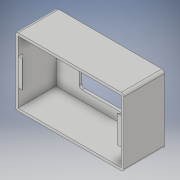
# Autodesk Inventor part: spodok
Saved by Autodesk Inventor 2019 (Build 230136000, 136)
## iProperties
Created: 2021-04-22
Part Number: spodok
Material: Všeobecné
Document SubType Name: Modeling
Designer: miko flosso
Density: 1 g/cm^3
Appearance: Výchozí
Author: miko flosso
Autodesk Inventor part; units mm, degrees
ref_plane "YZ Plane" through (0, 0, 0) normal (1, 0, 0) x (0, 1, 0)
ref_plane "XZ Plane" through (0, 0, 0) normal (0, 1, 0) x (-1, 0, 0)
sketch "Náčrt3" plane through (0, 0, 0) normal (0, 0, 1) x (1, 0, 0)
  line L0 (2, 0) -> (78, 0)
  line L1 (80, -2) -> (80, -48)
  line L2 (78, -50) -> (2, -50)
  line L3 (0, -48) -> (0, -2)
  arc A0 (2, 0) -> (0, -2) centre (2, -2) ccw
  arc A1 (0, -48) -> (2, -50) centre (2, -48) ccw
  arc A2 (80, -2) -> (78, 0) centre (78, -2) ccw
  arc A3 (78, -50) -> (80, -48) centre (78, -48) ccw
  point P0 (0, 0)
  point P1 (80, -50)
  point P2 (80, 0)
  point P3 (0, -50)
  dimension "d4" = 80
  dimension "d5" = 50
  dimension "d6" = 2
  constraints: 8 end point, 8 point on circle, 8 point on line, 8 tangent, 4 centre point, 3 equal radius, 2 parallel, 1 horizontal, 1 perpendicular
  measures "d4" distance of point (80, -50) point (0, -50)
  measures "d5" distance of point (80, 0) point (80, -50)
  measures "d6" radius of A0
extrude "Vysunutí2" add sketch "Náčrt3" along normal blind 30
shell "Skořepina1" thickness 2 removed faces 1 at (27.3333, -16.6667, 30)
sketch "Náčrt4" plane through (2, -48, 30) normal (1, 0, 0) x (0, 0, -1)
  line L0 (0.0823, 33) -> (3.0823, 33)
  line L1 (3.0823, 33) -> (3.0823, 13)
  line L2 (3.0823, 13) -> (0.0823, 13)
  line L3 (0.0823, 13) -> (0.0823, 33)
  point P0 (30, 48)
  dimension "d10" = 3
  dimension "d11" = 20
  dimension "d12" = 15
  constraints: 8 end point, 2 parallel, 1 horizontal, 1 perpendicular
  measures "d10" distance of L1.end L2.end
  measures "d11" distance of L0.end L1.end
  measures "d12" distance from line of point (30, 48) L0
extrude "Vysunutí3" add sketch "Náčrt4" along normal blind 3
chamfer "Zkosení1" distance 2.5 angle 45 1 edges at (5, -25, 26.9177)
ref_plane "Pracovní rovina2" through (40, -48, 0) normal (1, 0, 0) x (0, 0, -1)
mirror "Zrcadlit1" about plane through (40, -48, 0) normal (1, 0, 0) of "Vysunutí3", "Zkosení1"
sketch "Náčrt5" plane through (2, -48, 2) normal (0, 0, 1) x (1, 0, 0)
  line L0 (19.0725, 36.0953) -> (62.5669, 36.0953)
  line L1 (64.5669, 34.0953) -> (64.5669, 9.1748)
  line L2 (62.5669, 7.1748) -> (19.0725, 7.1748)
  line L3 (17.0725, 9.1748) -> (17.0725, 34.0953)
  arc A0 (19.0725, 36.0953) -> (17.0725, 34.0953) centre (19.0725, 34.0953) ccw
  arc A1 (17.0725, 9.1748) -> (19.0725, 7.1748) centre (19.0725, 9.1748) ccw
  arc A2 (64.5669, 34.0953) -> (62.5669, 36.0953) centre (62.5669, 34.0953) ccw
  arc A3 (62.5669, 7.1748) -> (64.5669, 9.1748) centre (62.5669, 9.1748) ccw
  point P0 (-2, 48)
  dimension "d19" = 2
  constraints: 8 end point, 8 point on circle, 8 tangent, 4 centre point, 3 equal radius, 2 parallel, 1 horizontal, 1 perpendicular
  measures "d19" radius of A0
extrude "Vysunutí4" cut sketch "Náčrt5" against normal blind 3
